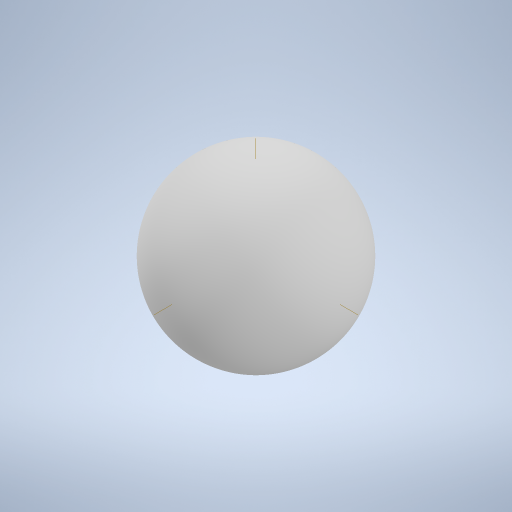
# Autodesk Inventor part: Sphere
Saved by Autodesk Inventor 2023.1 (Build 271208000, 208)
## iProperties
Created: 2023-01-19
Part Number: Sphere
Material: Generisch
Document SubType Name: Modeling
Designer: mehan
Density: 1 g/cm^3
Appearance: Vorgabe
Author: mehan
Autodesk Inventor part; units mm, degrees
ref_plane "YZ Plane" through (0, 0, 0) normal (1, 0, 0) x (0, 1, 0)
ref_plane "XZ Plane" through (0, 0, 0) normal (0, 1, 0) x (-1, 0, 0)
ref_plane "XY Plane" through (0, 0, 0) normal (0, 0, 1) x (1, 0, 0)
sketch "Skizze1" plane through (0, 0, 0) normal (0, 1, 0) x (-1, 0, 0)
  arc A0 (0, 50) -> (0, -50) centre (0, 0) ccw
  line L0 (0, 50) -> (0, -50)
  point P0 (-50, 0)
  dimension "d2" = 100
  constraints: 3 point on circle, 2 end point, 1 centre point, 1 coincident, 1 midpoint, 1 vertical
  measures "d2" diameter of point (-50, 0) point (0, 0)
revolve "Umdrehung1" add sketch "Skizze1" angle 360 about axis through (0, 0, 50) along (0, 0, -1)
